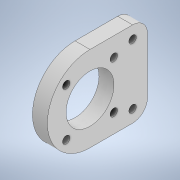
# Autodesk Inventor part: Soporte motor
Saved by Autodesk Inventor 2022 (Build 260153000, 153)
## iProperties
Created: 2022-02-20
Part Number: Soporte motor
Material: Generic
Document SubType Name: Modeling
Designer: juanp
Density: 1 g/cm^3
Appearance: Default
Author: juanp
Autodesk Inventor part; units mm, degrees
ref_plane "YZ Plane" through (0, 0, 0) normal (1, 0, 0) x (0, 1, 0)
ref_plane "XZ Plane" through (0, 0, 0) normal (0, 1, 0) x (-1, 0, 0)
ref_plane "XY Plane" through (0, 0, 0) normal (0, 0, 1) x (1, 0, 0)
sketch "Sketch1" plane through (0, 0, 0) normal (1, 0, 0) x (0, 1, 0)
  circle A0 centre (0, 0) radius 22.5 construction
  circle A1 centre (0, 0) radius 16.05
  circle A2 centre (0, 0) radius 28.5
  circle A3 centre (15.9099, 15.9099) radius 2.5
  line L0 (15.9099, 15.9099) -> (0, 0) construction
  circle A4 centre (-15.9099, 15.9099) radius 2.5
  circle A5 centre (-15.9099, -15.9099) radius 2.5
  circle A6 centre (15.9099, -15.9099) radius 2.5
  line L1 (28.5, 0) -> (28.5, -38.5)
  line L2 (28.5, -38.5) -> (-28.5, -38.5)
  line L3 (-28.5, -38.5) -> (-28.5, 0)
  line L4 (28.5, -18.5) -> (-28.5, -18.5)
  line L5 (-28.5, -28.5) -> (-20.1554, -28.5) construction
  line L6 (-20.1554, -28.5) -> (-11.8108, -28.5) construction
  line L7 (20.1554, -28.5) -> (28.5, -28.5) construction
  circle A7 centre (20.1554, -28.5) radius 2.5
  circle A8 centre (-20.1554, -28.5) radius 2.5
  line L8 (0, 0) -> (0, 13.3225) construction
  line L9 (-28.5, -28.5) -> (-20.1554, -28.5) construction
  line L10 (20.1554, -28.5) -> (16.456, -23.2691) construction
  point P0 (-17.3108, 22.6404)
  point P1 (-26.3306, -10.9065)
  point P2 (28.5, 0)
  dimension "d0" = 45
  dimension "d1" = 32.1
  dimension "d2" = 57
  dimension "d3" = 5
  dimension "d6" = 360
  dimension "d12" = 20
  dimension "d22" = 5
  dimension "d23" = 10
  dimension "d24" = 45
  dimension "d27" = 10
  dimension "d28" = 8.3446
  constraints: 22 end point, 8 centre point, 6 point on line, 5 coincident, 4 point on circle, 3 collinear, 2 horizontal, 2 perpendicular, 2 tangent, 2 vertical, 1 equal radius, 1 line through centre, 12 other
  measures "d1" diameter of A1
  measures "d2" diameter of A2
  measures "d3" diameter of A3
  measures "d12" distance between parallel lines of L2 L4
  measures "d22" diameter of A7
  measures "d23" distance between parallel lines of L2 L7
  measures "d24" angle of L0 L8
  measures "d27" distance edge to line of A2 L4
  measures "d28" distance of L7.start L7.end
extrude "Extrusion1" add sketch "Sketch1" along normal blind 10
fillet "Fillet1" radius 10 4 edges at (5, 28.5, -38.5) (5, -28.5, -38.5) (5, -28.5, 0) (5, 28.5, 0)
sketch "Sketch2" plane through (0, 0, 0) normal (-1, 0, 0) x (0, 0, 1)
  arc A0 (-38.5, -18.5) -> (-28.5, -28.5) centre (-28.5, -18.5) ccw projected
  line L0 (0, -28.5) -> (-28.5, -28.5) projected
  arc A1 (0, -28.5) -> (0, 28.5) centre (0, 0) ccw projected
  line L1 (-28.5, 28.5) -> (0, 28.5) projected
  arc A2 (-28.5, 28.5) -> (-38.5, 18.5) centre (-28.5, 18.5) ccw projected
  line L2 (-38.5, -18.5) -> (-38.5, 18.5) projected
  circle A3 centre (-28.5, 20.1554) radius 2.5 projected
  circle A4 centre (-28.5, -20.1554) radius 2.5 projected
  circle A5 centre (-15.9099, 15.9099) radius 2.5 projected
  circle A6 centre (-15.9099, -15.9099) radius 2.5 projected
  circle A7 centre (15.9099, -15.9099) radius 2.5 projected
  circle A8 centre (15.9099, 15.9099) radius 2.5 projected
  circle A9 centre (0, 0) radius 16.05 projected
  circle A10 centre (-15.9099, 15.9099) radius 2.5 projected
  circle A11 centre (-15.9099, 15.9099) radius 4.5
  circle A12 centre (-15.9099, -15.9099) radius 2.5 projected
  circle A13 centre (-15.9099, -15.9099) radius 4.5
  circle A14 centre (15.9099, -15.9099) radius 2.5 projected
  circle A15 centre (15.9099, -15.9099) radius 4.5
  circle A16 centre (15.9099, 15.9099) radius 2.5 projected
  circle A17 centre (15.9099, 15.9099) radius 4.5
  dimension "d29" = 9
  dimension "d30" = 9
  dimension "d31" = 9
  dimension "d32" = 9
  constraints: 4 centre point, 4 coincident
  measures "d29" diameter of A11
  measures "d30" diameter of A13
  measures "d31" diameter of A15
  measures "d32" diameter of A17
extrude "Extrusion2" cut sketch "Sketch2" against normal blind 5 contours A5 | A6 | A7 | A8 | A11 | A13 | A15 | A17
body "Solid1"
